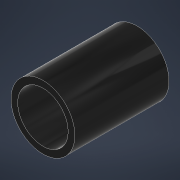
# Autodesk Inventor part: centerAxleBearingSpacer
Saved by Autodesk Inventor 2021.4 (Build 254397000, 397)
## iProperties
Created: 2022-03-02
Part Number: centerAxleBearingSpacer
Material: Generic
Document SubType Name: Modeling
Designer: jo_ki
Density: 1 g/cm^3
Appearance: Smooth - Black
Author: jo_ki
Autodesk Inventor part; units mm, degrees
ref_plane "YZ Plane" through (0, 0, 0) normal (1, 0, 0) x (0, 1, 0)
ref_plane "XZ Plane" through (0, 0, 0) normal (0, 1, 0) x (-1, 0, 0)
ref_plane "XY Plane" through (0, 0, 0) normal (0, 0, 1) x (1, 0, 0)
sketch "Sketch1" plane through (0, 0, 0) normal (0, 1, 0) x (-1, 0, 0)
  line L0 (-9.5, 0) -> (-7.5, 0)
  line L1 (-7.5, 0) -> (-7.5, -30)
  line L2 (-7.5, -30) -> (-9.5, -30)
  line L3 (-9.5, -30) -> (-9.5, 0)
  line L4 (0, -36) -> (0, 6) projected
  point P0 (0, 0)
  dimension "d0" = 2
  dimension "d1" = 30
  dimension "d3" = 9.5
  constraints: 8 end point, 2 parallel, 1 horizontal, 1 perpendicular, 1 point on line
  measures "d0" distance between parallel lines of L1 L3
  measures "d1" distance from line of L0.end L2
  measures "d3" distance from line of point (0, 0) L3
revolve "Revolution1" add sketch "Sketch1" angle 360 about axis through (0, 0, -10) along (0, 0, 1)
body "Solid1"
